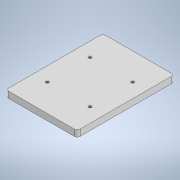
# Autodesk Inventor part: feste
Saved by Autodesk Inventor 2022 (Build 260153000, 153)
## iProperties
Created: 2022-04-28
Part Number: feste
Material: Generic
Document SubType Name: Modeling
Designer: eivin
Density: 1 g/cm^3
Appearance: Default
Author: eivin
Autodesk Inventor part; units mm, degrees
ref_plane "YZ Plane" through (0, 0, 0) normal (1, 0, 0) x (0, 1, 0)
ref_plane "XZ Plane" through (0, 0, 0) normal (0, 1, 0) x (-1, 0, 0)
ref_plane "XY Plane" through (0, 0, 0) normal (0, 0, 1) x (1, 0, 0)
sketch "Sketch1" plane through (0, 0, 0) normal (0, 1, 0) x (-1, 0, 0)
  line L0 (-25, -34) -> (25, -34)
  line L1 (25, -34) -> (25, 34)
  line L2 (25, 34) -> (-25, 34)
  line L3 (-25, 34) -> (-25, -34)
  line L4 (-25, -34) -> (25, 34) construction
  line L5 (25, -34) -> (-25, 34) construction
  point P0 (0, 0)
  dimension "d0" = 50
  dimension "d1" = 68
  constraints: 12 end point, 2 midpoint, 2 parallel, 1 horizontal, 1 perpendicular
  measures "d0" distance of L2.end L1.end
  measures "d1" distance of L1.end L0.end
extrude "Extrusion1" add sketch "Sketch1" along normal blind 4.5
sketch "Sketch2" plane through (0, 4.5, 0) normal (0, 1, 0) x (1, 0, 0)
  circle A0 centre (-15, 15) radius 1
  circle A1 centre (15, 15) radius 1
  circle A2 centre (15, -15) radius 1
  circle A3 centre (-15, -15) radius 1
  point P0 (0, 0)
  dimension "d4" = 2
  dimension "d5" = 2
  dimension "d6" = 2
  dimension "d7" = 2
  constraints: 4 centre point
  measures "d4" diameter of A0
  measures "d5" diameter of A1
  measures "d6" diameter of A2
  measures "d7" diameter of A3
extrude "Extrusion2" cut sketch "Sketch2" against normal blind 4.5
sketch "Sketch3" plane through (0, 0, 0) normal (0, -1, 0) x (1, 0, 0)
  circle A0 centre (15, 15) radius 2.5
  circle A1 centre (-15, 15) radius 2.5
  circle A2 centre (-15, -15) radius 2.5
  circle A3 centre (15, -15) radius 2.5
  circle A4 centre (15, -15) radius 1
  circle A5 centre (15, 15) radius 1 projected
  circle A6 centre (15, 15) radius 1
  circle A7 centre (-15, 15) radius 1 projected
  circle A8 centre (-15, 15) radius 1
  circle A9 centre (-15, -15) radius 1
  point P0 (0, 0)
  dimension "d10" = 5
  dimension "d11" = 5
  dimension "d12" = 5
  constraints: 8 centre point, 6 coincident
  measures "d10" diameter of A0
  measures "d11" diameter of A1
  measures "d12" diameter of A2
extrude "Extrusion3" add sketch "Sketch3" along normal blind 5
fillet "Fillet1" radius 2 4 edges at (-25, 2.25, 34) (25, 2.25, 34) (25, 2.25, -34) (-25, 2.25, -34)
fillet "Fillet2" radius 1 4 edges at (12.5, 0, -15) (12.5, 0, 15) (-17.5, 0, -15) (-17.5, 0, 15)
body "Solid1"
